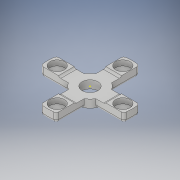
# Autodesk Inventor part: Disk-3
Saved by Autodesk Inventor 2019 (Build 230136000, 136)
## iProperties
Created: 2020-02-07
Part Number: Disk-3
Material: Generic
Document SubType Name: Modeling
Designer: gfb14170
Density: 1 g/cm^3
Appearance: Default
Author: gfb14170
Autodesk Inventor part; units mm, degrees
ref_plane "YZ Plane" through (0, 0, 0) normal (1, 0, 0) x (0, 1, 0)
ref_plane "XZ Plane" through (0, 0, 0) normal (0, 1, 0) x (-1, 0, 0)
ref_plane "XY Plane" through (0, 0, 0) normal (0, 0, 1) x (1, 0, 0)
sketch "Sketch1" plane through (0, 0, 0) normal (0, 1, 0) x (-1, 0, 0)
  circle A0 centre (0, 0) radius 3
  circle A1 centre (0, 0) radius 6 construction
  circle A2 centre (0, 0) radius 16 construction
  line L0 (-3, 15.7162) -> (-3, 5.1962)
  line L1 (3, 5.2197) -> (3, 15.7162)
  arc A3 (3, 15.7162) -> (-3, 15.7162) centre (0, 0) ccw
  line L2 (-5.2197, 3) -> (-15.7162, 3)
  arc A4 (-15.7162, 3) -> (-15.7162, -3) centre (0, 0) ccw
  line L3 (-15.7162, -3) -> (-5.1962, -3)
  line L4 (-3, -5.2197) -> (-3, -15.7162)
  arc A5 (-3, -15.7162) -> (3, -15.7162) centre (0, 0) ccw
  line L5 (3, -15.7162) -> (3, -5.1962)
  line L6 (5.2197, -3) -> (15.7162, -3)
  arc A6 (15.7162, -3) -> (15.7162, 3) centre (0, 0) ccw
  line L7 (15.7162, 3) -> (5.1962, 3)
  arc A7 (5.1962, 3) -> (3, 5.2197) centre (-0.2008, -0.1435) ccw
  arc A8 (3, -5.1962) -> (5.2197, -3) centre (-0.1229, 0.18) ccw
  arc A9 (-3, 5.1962) -> (-5.2197, 3) centre (0.1893, -0.2471) ccw
  arc A10 (-5.1962, -3) -> (-3, -5.2197) centre (0.2474, 0.1896) ccw
  dimension "d1" = 12
  dimension "d0" = 6
  dimension "d2" = 32
  dimension "d3" = 3
  dimension "d4" = 3
  dimension "d8" = 360
  constraints: 18 point on circle, 16 end point, 10 centre point, 5 coincident, 1 concentric, 1 parallel, 34 other
  measures "d0" diameter of A0
  measures "d2" diameter of A2
  measures "d3" distance from line of point (0, 0) L1
  measures "d4" distance from line of point (0, 0) L0
extrude "Extrusion1" add sketch "Sketch1" along normal blind 3
sketch "Sketch2" plane through (0, 3, 0) normal (0, 1, 0) x (1, 0, 0)
  circle A0 centre (0, -12.5) radius 2.75
  circle A1 centre (12.5, 0) radius 2.75
  circle A2 centre (0, 12.5) radius 2.75
  circle A3 centre (-12.5, 0) radius 2.75
  point P0 (0, 0)
  point P1 (0, 12.5)
  point P2 (-12.5, 0)
  dimension "d12" = 5.5
  dimension "d13" = 12.5
  dimension "d16" = 360
  dimension "d18" = 0
  dimension "d24" = 360
  constraints: 4 centre point, 14 other
  measures "d12" diameter of A0
  measures "d13" distance of point (0, 0) A0.centre
  measures "d18" horizontal distance of point (0, 0) A0.centre
sketch "Sketch3" plane through (0, 3, 0) normal (0, 1, 0) x (1, 0, 0)
  point P0 (0, 0)
extrude "Extrusion2" cut sketch "Sketch2" against normal blind 1.5
sketch "Sketch4" plane through (0, 3, 0) normal (0, 1, 0) x (1, 0, 0)
  circle A0 centre (0, 12.5) radius 2.75 projected
  circle A1 centre (0, -12.5) radius 2.75 projected
  circle A2 centre (12.5, 0) radius 2.75 projected
  circle A3 centre (-12.5, 0) radius 2.75 projected
  circle A4 centre (0, 0) radius 3 projected
  line L0 (-3, -5.2197) -> (-3, -15.7162) projected
  arc A5 (-3, -15.7162) -> (3, -15.7162) centre (0, 0) ccw projected
  line L1 (3, -15.7162) -> (3, -5.1962) projected
  arc A6 (3, -5.1962) -> (5.2197, -3) centre (-0.1893, 0.2471) ccw projected
  line L2 (5.2197, -3) -> (15.7162, -3) projected
  arc A7 (15.7162, -3) -> (15.7162, 3) centre (0, 0) ccw projected
  line L3 (15.7162, 3) -> (5.1962, 3) projected
  arc A8 (5.1962, 3) -> (3, 5.2197) centre (-0.2474, -0.1896) ccw projected
  line L4 (3, 5.2197) -> (3, 15.7162) projected
  arc A9 (3, 15.7162) -> (-3, 15.7162) centre (0, 0) ccw projected
  line L5 (-3, 15.7162) -> (-3, 5.1962) projected
  arc A10 (-3, 5.1962) -> (-5.2197, 3) centre (0.1229, -0.18) ccw projected
  line L6 (-5.2197, 3) -> (-15.7162, 3) projected
  arc A11 (-15.7162, 3) -> (-15.7162, -3) centre (0, 0) ccw projected
  line L7 (-15.7162, -3) -> (-5.1962, -3) projected
  arc A12 (-5.1962, -3) -> (-3, -5.2197) centre (0.2008, 0.1435) ccw projected
  arc A13 (15.7162, -3) -> (15.7162, 3) centre (0, 0) ccw
  line L8 (5.2197, -3) -> (15.7162, -3) projected
  line L9 (15.7162, 3) -> (5.1962, 3) projected
  line L10 (15.7162, -3) -> (9, -3)
  line L11 (9, -3) -> (9, 3)
  line L12 (9, 3) -> (15.7162, 3)
  line L13 (3, 9) -> (-3, 9)
  line L14 (-9, 3) -> (-9, -3)
  line L15 (-3, -15.7162) -> (-3, -5.2197) projected
  arc A14 (-3, -15.7162) -> (3, -15.7162) centre (0, -0.0001) ccw
  arc A15 (-3, -15.7162) -> (3, -15.7162) centre (0, 0) ccw projected
  arc A16 (-3, -15.7162) -> (3, -15.7162) centre (0, -0.0001) ccw
  line L16 (-3, -5.2197) -> (-3, -15.7162) projected
  line L17 (-3, -15.7162) -> (-3, -9)
  line L18 (3, -5.1962) -> (3, -15.7162) projected
  line L19 (3, -9) -> (3, -15.7162)
  line L20 (3, 15.7162) -> (3, 9)
  line L21 (3, 9) -> (-3, 9)
  arc A17 (3, 15.7162) -> (-3, 15.7162) centre (0, 0) ccw
  line L22 (-3, 9) -> (-3, 15.7162)
  line L23 (-15.7162, 3) -> (-9, 3)
  line L24 (-9, 3) -> (-9, -3)
  arc A18 (-15.7162, 3) -> (-15.7162, -3) centre (0, 0) ccw
  line L25 (-9, -3) -> (-15.7162, -3)
  line L26 (-3, -15.7162) -> (-3, -9)
  line L27 (-3, -9) -> (3, -9)
  arc A19 (-3, -15.7162) -> (3, -15.7162) centre (0, 0) ccw
  line L28 (3, -9) -> (3, -15.7162)
  arc A20 (3, 15.7162) -> (-3, 15.7162) centre (0, 0) ccw
  line L29 (3, 5.2197) -> (3, 15.7162) projected
  line L30 (3, 15.7162) -> (-3, 15.7162)
  line L31 (-3, 15.7162) -> (-3, 9)
  line L32 (-3, 9) -> (3, 9)
  line L33 (3, 9) -> (3, 15.7162)
  line L34 (-15.7162, -3) -> (-5.1962, -3) projected
  arc A21 (-15.7162, 3) -> (-15.7162, -3) centre (0, 0) ccw
  line L35 (-15.7162, -3) -> (-9, -3)
  line L36 (-9, -3) -> (-9, 3)
  line L37 (-9, 3) -> (-15.7162, 3)
  line L38 (-15.7162, 3) -> (-15.7162, -3)
  arc A22 (-3, -15.7162) -> (3, -15.7162) centre (0, 0) ccw
  line L39 (3, -15.7162) -> (-3, -15.7162)
  line L40 (-3, -15.7162) -> (-3, -9)
  line L41 (-3, -9) -> (3, -9)
  line L42 (3, -9) -> (3, -15.7162)
  point P0 (0, 0)
  dimension "d0" = 6
  dimension "d1" = 12
  dimension "d2" = 32
  dimension "d3" = 3
  dimension "d4" = 3
  dimension "d8" = 360
  dimension "d28" = 3.5
  dimension "d35" = 360
  constraints: 56 end point, 18 point on circle, 9 centre point, 7 parallel, 4 horizontal, 4 perpendicular, 1 collinear, 1 concentric, 1 point on line, 41 other
  measures "d28" distance from line of L11 A2.centre
extrude "Extrusion3" add sketch "Sketch4" along normal blind 0.5 contours L27 L1 L39 L0 | L39 A5 | L7 L38 L6 L14 | A11 L38 | L11 L3 A7 L2 | L5 L30 L4 L13 | A9 L30
fillet "Fillet1" radius 1 4 edges at (16, 0, 0) (0, 0, 16) (-16, 0, 0) (0, 0, -16)
fillet "Fillet2" radius 1 4 edges at (9, 3, 0) (0, 3, 9) (-9, 3, 0) (0, 3, -9)
fillet "Fillet3" radius 1 24 edges at (15.4161, 0.2911, -3) (9.9465, 0, -3) (15.7162, 2.25, -3) (15.4161, 0.2911, 3) (9.9583, 0, 3) (15.7162, 2.25, 3) (3, 0.2911, -15.4161) (3, 0, -9.9583) (3, 2.25, -15.7162) (-3, 0.2911, -15.4161) (-3, 0, -9.9465) (-3, 2.25, -15.7162) (-15.4161, 0.2911, -3) (-9.9583, 0, -3) (-15.7162, 2.25, -3) (3, 2.25, 15.7162) (3, 0, 9.9465) (3, 0.2911, 15.4161) (-3, 0.2911, 15.4161) (-3, 2.25, 15.7162) (-3, 0, 9.9583) (-15.4161, 0.2911, 3) (-15.7162, 2.25, 3) (-9.9465, 0, 3)
equation "\"d4\" = d3"
body "Solid1"
